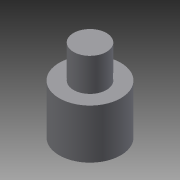
# Autodesk Inventor part: gear motor
Saved by Autodesk Inventor 2015 (Build 190159000, 159)
## iProperties
Created: 2012-08-16
Part Number: gear motor
Material: Generic
Document SubType Name: Modeling
Designer: idle-rug
Density: 1 g/cm^3
Appearance: Default
Author: idle-rug
Autodesk Inventor part; units mm, degrees
ref_plane "YZ Plane" through (0, 0, 0) normal (1, 0, 0) x (0, 1, 0)
ref_plane "XZ Plane" through (0, 0, 0) normal (0, 1, 0) x (-1, 0, 0)
sketch "Sketch1" plane through (0, 0, 0) normal (0, 0, 1) x (1, 0, 0)
  circle A0 centre (0, 0) radius 5.6
  dimension "d0" = 11.2
  constraints: 1 centre point, 1 coincident
  measures "d0" diameter of A0
extrude "Extrusion1" add sketch "Sketch1" against normal blind 9
ref_plane "Work Plane1" through (-5.6, 5.6, 0) normal (0, 1, 0) x (1, 0, 0)
sketch "Sketch3" plane through (-5.6, 5.6, 0) normal (0, 1, 0) x (1, 0, 0)
  circle A0 centre (5.6, 4.5) radius 1.2
  point P0 (5.6, 0)
  dimension "d9" = 2.4
  constraints: 1 centre point
  measures "d9" diameter of A0
hole "Hole1" at (0, 5.6, -4.5) direction (0, -1, 0) diameter 2.459 depth 5.6 thread size "M3x0.5" designation "M3" class "6H" standard "GB Metric profile"
sketch "Sketch4" plane through (0, 0, 0) normal (0, 0, 1) x (1, 0, 0)
  circle A0 centre (0, 0) radius 5.6 projected
  circle A1 centre (0, 0) radius 3
  dimension "d17" = 6
  constraints: 1 centre point, 1 coincident
  measures "d17" diameter of A1
extrude "Extrusion3" add sketch "Sketch4" along normal blind 6 contours A1
body "Solid1"
